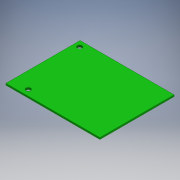
# Autodesk Inventor part: モタドラ
Saved by Autodesk Inventor 2018 (Build 220112000, 112)
## iProperties
Created: 2018-08-16
Part Number: モタドラ
Material: 一般
Document SubType Name: Modeling
Designer: shun2
Density: 1 g/cm^3
Appearance: 濃い緑
Author: shun2
Autodesk Inventor part; units mm, degrees
(part 1 of 2)
ref_plane "YZ Plane" through (0, 0, 0) normal (1, 0, 0) x (0, 1, 0)
ref_plane "XZ Plane" through (0, 0, 0) normal (0, 1, 0) x (-1, 0, 0)
ref_plane "XY Plane" through (0, 0, 0) normal (0, 0, 1) x (1, 0, 0)
sketch "スケッチ1" plane through (0, 0, 0) normal (0, 0, 1) x (1, 0, 0)
  line L0 (65.024, -2.794) -> (65.024, -0.3175)
  line L1 (0, -2.794) -> (0, -0.3175)
  line L2 (37.2085, -2.54) -> (65.024, -2.54)
  line L3 (0, -2.54) -> (27.0027, -2.54)
  line L4 (63.5, -2.032) -> (65.024, -2.54)
  line L5 (63.5, -3.048) -> (65.024, -2.54)
  line L6 (0, -2.54) -> (1.524, -3.048)
  line L7 (0, -2.54) -> (1.524, -2.032)
  line L8 (-2.794, 51.308) -> (-0.3175, 51.308)
  line L9 (-2.794, 0) -> (-0.3175, 0)
  line L10 (-2.54, 30.3505) -> (-2.54, 51.308)
  line L11 (-2.54, 0) -> (-2.54, 20.1447)
  line L12 (-3.048, 49.784) -> (-2.54, 51.308)
  line L13 (-2.54, 51.308) -> (-2.032, 49.784)
  line L14 (-2.54, 0) -> (-2.032, 1.524)
  line L15 (-3.048, 1.524) -> (-2.54, 0)
  line L16 (0, 0) -> (0, 51.308)
  line L17 (0, 51.308) -> (65.024, 51.308)
  line L18 (65.024, 0) -> (65.024, 51.308)
  line L19 (0, 0) -> (65.024, 0)
  line L20 (2.2225, 47.244) -> (5.3975, 47.244)
  line L21 (3.81, 45.6565) -> (3.81, 48.8315)
  line L22 (9.8425, 4.064) -> (13.0175, 4.064)
  line L23 (11.43, 2.4765) -> (11.43, 5.6515)
  line L24 (1.016, 24.384) -> (2.032, 24.384)
  line L25 (1.524, 23.876) -> (1.524, 24.892)
  line L26 (1.016, 21.844) -> (2.032, 21.844)
  line L27 (1.524, 21.336) -> (1.524, 22.352)
  line L28 (1.016, 19.304) -> (2.032, 19.304)
  line L29 (1.524, 18.796) -> (1.524, 19.812)
  line L30 (1.016, 16.764) -> (2.032, 16.764)
  line L31 (1.524, 16.256) -> (1.524, 17.272)
  line L32 (1.016, 14.224) -> (2.032, 14.224)
  line L33 (1.524, 13.716) -> (1.524, 14.732)
  line L34 (1.016, 32.004) -> (2.032, 32.004)
  line L35 (1.524, 31.496) -> (1.524, 32.512)
  line L36 (1.016, 29.464) -> (2.032, 29.464)
  line L37 (1.524, 28.956) -> (1.524, 29.972)
  line L38 (1.016, 26.924) -> (2.032, 26.924)
  line L39 (1.524, 26.416) -> (1.524, 27.432)
  line L40 (1.016, 1.524) -> (2.032, 1.524)
  line L41 (1.524, 1.016) -> (1.524, 2.032)
  line L42 (1.016, 4.064) -> (2.032, 4.064)
  line L43 (1.524, 3.556) -> (1.524, 4.572)
  line L44 (1.016, 6.604) -> (2.032, 6.604)
  line L45 (1.524, 6.096) -> (1.524, 7.112)
  line L46 (1.016, 9.144) -> (2.032, 9.144)
  line L47 (1.524, 8.636) -> (1.524, 9.652)
  line L48 (1.016, 11.684) -> (2.032, 11.684)
  line L49 (1.524, 11.176) -> (1.524, 12.192)
  line L50 (8.382, 47.244) -> (9.398, 47.244)
  line L51 (8.89, 46.736) -> (8.89, 47.752)
  line L52 (8.382, 44.704) -> (9.398, 44.704)
  line L53 (8.89, 44.196) -> (8.89, 45.212)
  line L54 (10.922, 47.244) -> (11.938, 47.244)
  line L55 (11.43, 46.736) -> (11.43, 47.752)
  line L56 (10.922, 44.704) -> (11.938, 44.704)
  line L57 (11.43, 44.196) -> (11.43, 45.212)
  line L58 (13.462, 47.244) -> (14.478, 47.244)
  line L59 (13.97, 46.736) -> (13.97, 47.752)
  line L60 (13.462, 44.704) -> (14.478, 44.704)
  line L61 (13.97, 44.196) -> (13.97, 45.212)
  line L62 (16.002, 47.244) -> (17.018, 47.244)
  line L63 (16.51, 46.736) -> (16.51, 47.752)
  line L64 (16.002, 44.704) -> (17.018, 44.704)
  line L65 (16.51, 44.196) -> (16.51, 45.212)
  line L66 (10.922, 39.497) -> (11.938, 39.497)
  line L67 (11.43, 38.989) -> (11.43, 40.005)
  line L68 (10.922, 36.957) -> (11.938, 36.957)
  line L69 (11.43, 36.449) -> (11.43, 37.465)
  line L70 (13.462, 39.497) -> (14.478, 39.497)
  line L71 (13.97, 38.989) -> (13.97, 40.005)
  line L72 (13.462, 36.957) -> (14.478, 36.957)
  line L73 (13.97, 36.449) -> (13.97, 37.465)
  line L74 (16.002, 39.497) -> (17.018, 39.497)
  line L75 (16.51, 38.989) -> (16.51, 40.005)
  line L76 (16.002, 36.957) -> (17.018, 36.957)
  line L77 (16.51, 36.449) -> (16.51, 37.465)
  line L78 (18.542, 39.497) -> (19.558, 39.497)
  line L79 (19.05, 38.989) -> (19.05, 40.005)
  line L80 (18.542, 36.957) -> (19.558, 36.957)
  line L81 (19.05, 36.449) -> (19.05, 37.465)
  line L82 (19.431, 5.207) -> (20.447, 5.207)
  line L83 (19.939, 4.699) -> (19.939, 5.715)
  line L84 (19.431, 10.2057) -> (20.447, 10.2057)
  line L85 (19.939, 9.7003) -> (19.939, 10.7137)
  line L86 (19.431, 5.207) -> (20.447, 5.207)
  line L87 (19.939, 4.699) -> (19.939, 5.715)
  line L88 (19.431, 8.7071) -> (20.447, 8.7071)
  line L89 (19.939, 8.1991) -> (19.939, 9.2151)
  line L90 (20.066, 14.605) -> (21.082, 14.605)
  line L91 (20.574, 14.097) -> (20.574, 15.113)
  line L92 (22.606, 14.605) -> (23.622, 14.605)
  line L93 (23.114, 14.097) -> (23.114, 15.113)
  line L94 (26.289, 6.858) -> (27.305, 6.858)
  line L95 (26.797, 6.35) -> (26.797, 7.366)
  line L96 (26.289, 9.398) -> (27.305, 9.398)
  line L97 (26.797, 8.89) -> (26.797, 9.906)
  line L98 (26.289, 16.3347) -> (27.305, 16.3347)
  line L99 (26.797, 15.8267) -> (26.797, 16.8427)
  line L100 (25.781, 36.703) -> (26.797, 36.703)
  line L101 (26.289, 36.195) -> (26.289, 37.211)
  line L102 (23.241, 36.703) -> (24.257, 36.703)
  line L103 (23.749, 36.195) -> (23.749, 37.211)
  line L104 (25.4, 39.624) -> (26.416, 39.624)
  line L105 (25.908, 39.116) -> (25.908, 40.132)
  line L106 (59.4868, 28.1813) -> (61.6712, 28.1813)
  line L107 (60.579, 27.0891) -> (60.579, 29.2735)
  line L108 (59.4868, 23.1826) -> (61.6712, 23.1826)
  line L109 (60.579, 22.0904) -> (60.579, 24.2748)
  line L110 (59.4868, 13.1826) -> (61.6712, 13.1826)
  line L111 (60.579, 12.0904) -> (60.579, 14.2748)
  line L112 (59.4868, 18.1813) -> (61.6712, 18.1813)
  line L113 (60.579, 17.0891) -> (60.579, 19.2735)
  line L114 (59.4868, 33.1826) -> (61.6712, 33.1826)
  line L115 (60.579, 32.0904) -> (60.579, 34.2748)
  line L116 (59.4868, 38.1813) -> (61.6712, 38.1813)
  line L117 (60.579, 37.0891) -> (60.579, 39.2735)
  line L118 (61.976, 19.304) -> (62.992, 19.304)
  line L119 (62.484, 18.796) -> (62.484, 19.812)
  line L120 (61.976, 21.844) -> (62.992, 21.844)
  line L121 (62.484, 21.336) -> (62.484, 22.352)
  line L122 (61.976, 24.384) -> (62.992, 24.384)
  line L123 (62.484, 23.876) -> (62.484, 24.892)
  line L124 (61.976, 26.924) -> (62.992, 26.924)
  line L125 (62.484, 26.416) -> (62.484, 27.432)
  line L126 (61.976, 39.624) -> (62.992, 39.624)
  line L127 (62.484, 39.116) -> (62.484, 40.132)
  line L128 (61.976, 37.084) -> (62.992, 37.084)
  line L129 (62.484, 36.576) -> (62.484, 37.592)
  line L130 (61.976, 34.544) -> (62.992, 34.544)
  line L131 (62.484, 34.036) -> (62.484, 35.052)
  line L132 (61.976, 32.004) -> (62.992, 32.004)
  line L133 (62.484, 31.496) -> (62.484, 32.512)
  line L134 (61.976, 29.464) -> (62.992, 29.464)
  line L135 (62.484, 28.956) -> (62.484, 29.972)
  line L136 (61.976, 16.764) -> (62.992, 16.764)
  line L137 (62.484, 16.256) -> (62.484, 17.272)
  line L138 (61.976, 14.224) -> (62.992, 14.224)
  line L139 (62.484, 13.716) -> (62.484, 14.732)
  line L140 (61.976, 11.684) -> (62.992, 11.684)
  line L141 (62.484, 11.176) -> (62.484, 12.192)
  line L142 (54.61, 4.318) -> (55.626, 4.318)
  line L143 (55.118, 3.81) -> (55.118, 4.826)
  line L144 (54.61, 6.858) -> (55.626, 6.858)
  line L145 (55.118, 6.35) -> (55.118, 7.366)
  line L146 (57.15, 4.318) -> (58.166, 4.318)
  line L147 (57.658, 3.81) -> (57.658, 4.826)
  line L148 (57.15, 6.858) -> (58.166, 6.858)
  line L149 (57.658, 6.35) -> (57.658, 7.366)
  line L150 (25.908, 49.784) -> (26.924, 49.784)
  line L151 (26.416, 49.276) -> (26.416, 50.292)
  line L152 (18.288, 49.784) -> (19.304, 49.784)
  line L153 (18.796, 49.276) -> (18.796, 50.292)
  line L154 (28.448, 49.784) -> (29.464, 49.784)
  line L155 (28.956, 49.276) -> (28.956, 50.292)
  line L156 (32.512, 1.524) -> (33.528, 1.524)
  line L157 (33.02, 1.016) -> (33.02, 2.032)
  line L158 (30.988, 49.784) -> (32.004, 49.784)
  line L159 (31.496, 49.276) -> (31.496, 50.292)
  line L160 (33.528, 49.784) -> (34.544, 49.784)
  line L161 (34.036, 49.276) -> (34.036, 50.292)
  line L162 (36.068, 49.784) -> (37.084, 49.784)
  line L163 (36.576, 49.276) -> (36.576, 50.292)
  line L164 (38.608, 49.784) -> (39.624, 49.784)
  line L165 (39.116, 49.276) -> (39.116, 50.292)
  line L166 (41.148, 49.784) -> (42.164, 49.784)
  line L167 (41.656, 49.276) -> (41.656, 50.292)
  line L168 (45.212, 49.784) -> (46.228, 49.784)
  line L169 (45.72, 49.276) -> (45.72, 50.292)
  line L170 (47.752, 49.784) -> (48.768, 49.784)
  line L171 (48.26, 49.276) -> (48.26, 50.292)
  line L172 (50.292, 49.784) -> (51.308, 49.784)
  line L173 (50.8, 49.276) -> (50.8, 50.292)
  line L174 (52.832, 49.784) -> (53.848, 49.784)
  line L175 (53.34, 49.276) -> (53.34, 50.292)
  line L176 (55.372, 49.784) -> (56.388, 49.784)
  line L177 (55.88, 49.276) -> (55.88, 50.292)
  line L178 (57.912, 49.784) -> (58.928, 49.784)
  line L179 (58.42, 49.276) -> (58.42, 50.292)
  line L180 (60.452, 49.784) -> (61.468, 49.784)
  line L181 (60.96, 49.276) -> (60.96, 50.292)
  line L182 (62.992, 49.784) -> (64.008, 49.784)
  line L183 (63.5, 49.276) -> (63.5, 50.292)
  line L184 (35.052, 1.524) -> (36.068, 1.524)
  line L185 (35.56, 1.016) -> (35.56, 2.032)
  line L186 (37.592, 1.524) -> (38.608, 1.524)
  line L187 (38.1, 1.016) -> (38.1, 2.032)
  line L188 (40.132, 1.524) -> (41.148, 1.524)
  line L189 (40.64, 1.016) -> (40.64, 2.032)
  line L190 (42.672, 1.524) -> (43.688, 1.524)
  line L191 (43.18, 1.016) -> (43.18, 2.032)
  line L192 (45.212, 1.524) -> (46.228, 1.524)
  line L193 (45.72, 1.016) -> (45.72, 2.032)
  line L194 (50.292, 1.524) -> (51.308, 1.524)
  line L195 (50.8, 1.016) -> (50.8, 2.032)
  line L196 (52.832, 1.524) -> (53.848, 1.524)
  line L197 (53.34, 1.016) -> (53.34, 2.032)
  line L198 (55.372, 1.524) -> (56.388, 1.524)
  line L199 (55.88, 1.016) -> (55.88, 2.032)
  line L200 (57.912, 1.524) -> (58.928, 1.524)
  line L201 (58.42, 1.016) -> (58.42, 2.032)
  line L202 (60.452, 1.524) -> (61.468, 1.524)
  line L203 (60.96, 1.016) -> (60.96, 2.032)
  line L204 (62.992, 1.524) -> (64.008, 1.524)
  line L205 (63.5, 1.016) -> (63.5, 2.032)
  line L206 (23.368, 49.784) -> (24.384, 49.784)
  line L207 (23.876, 49.276) -> (23.876, 50.292)
  line L208 (20.828, 49.784) -> (21.844, 49.784)
  line L209 (21.336, 49.276) -> (21.336, 50.292)
  line L210 (27.432, 1.524) -> (28.448, 1.524)
  line L211 (27.94, 1.016) -> (27.94, 2.032)
  line L212 (29.972, 1.524) -> (30.988, 1.524)
  line L213 (30.48, 1.016) -> (30.48, 2.032)
  line L214 (49.3395, 25.654) -> (49.7205, 25.654)
  line L215 (49.53, 25.4635) -> (49.53, 25.8445)
  line L216 (50.7365, 25.654) -> (51.1175, 25.654)
  line L217 (50.927, 25.4635) -> (50.927, 25.8445)
  line L218 (49.8475, 26.416) -> (50.2285, 26.416)
  line L219 (50.038, 26.2255) -> (50.038, 26.6065)
  line L220 (48.8315, 26.416) -> (49.2125, 26.416)
  line L221 (49.022, 26.2255) -> (49.022, 26.6065)
  line L222 (48.3235, 25.654) -> (48.7045, 25.654)
  line L223 (48.514, 25.4635) -> (48.514, 25.8445)
  line L224 (29.0195, 35.4813) -> (29.4005, 35.4813)
  line L225 (29.21, 35.2908) -> (29.21, 35.6718)
  line L226 (38.9255, 33.528) -> (39.3065, 33.528)
  line L227 (39.116, 33.3375) -> (39.116, 33.7185)
  line L228 (25.5905, 27.051) -> (25.9715, 27.051)
  line L229 (25.781, 26.8605) -> (25.781, 27.2415)
  line L230 (28.1305, 26.035) -> (28.5115, 26.035)
  line L231 (28.321, 25.8445) -> (28.321, 26.2255)
  line L232 (28.1305, 27.051) -> (28.5115, 27.051)
  line L233 (28.321, 26.8605) -> (28.321, 27.2415)
  line L234 (27.2415, 22.479) -> (27.6225, 22.479)
  line L235 (27.432, 22.2885) -> (27.432, 22.6695)
  line L236 (28.1305, 28.067) -> (28.5115, 28.067)
  line L237 (28.321, 27.8765) -> (28.321, 28.2575)
  line L238 (6.1595, 12.954) -> (6.5405, 12.954)
  line L239 (6.35, 12.7635) -> (6.35, 13.1445)
  line L240 (2.9591, 28.321) -> (3.3401, 28.321)
  line L241 (3.1496, 28.1305) -> (3.1496, 28.5115)
  line L242 (5.1435, 12.954) -> (5.5245, 12.954)
  line L243 (5.334, 12.7635) -> (5.334, 13.1445)
  line L244 (6.6675, 15.113) -> (7.0485, 15.113)
  line L245 (6.858, 14.9225) -> (6.858, 15.3035)
  line L246 (11.8745, 11.557) -> (12.2555, 11.557)
  line L247 (12.065, 11.3665) -> (12.065, 11.7475)
  line L248 (12.1285, 50.038) -> (12.5095, 50.038)
  line L249 (12.319, 49.8475) -> (12.319, 50.2285)
  line L250 (21.1455, 41.402) -> (21.5265, 41.402)
  line L251 (21.336, 41.2115) -> (21.336, 41.5925)
  line L252 (20.259, 43.18) -> (20.64, 43.18)
  line L253 (20.4495, 42.9895) -> (20.4495, 43.3705)
  line L254 (49.8475, 27.94) -> (50.2285, 27.94)
  line L255 (50.038, 27.7495) -> (50.038, 28.1305)
  line L256 (48.8315, 27.94) -> (49.2125, 27.94)
  line L257 (49.022, 27.7495) -> (49.022, 28.1305)
  line L258 (49.8475, 24.892) -> (50.2285, 24.892)
  line L259 (50.038, 24.7015) -> (50.038, 25.0825)
  line L260 (60.6425, 30.226) -> (61.0235, 30.226)
  line L261 (60.833, 30.0355) -> (60.833, 30.4165)
  line L262 (59.1185, 30.226) -> (59.4995, 30.226)
  line L263 (59.309, 30.0355) -> (59.309, 30.4165)
  line L264 (26.858, 43.18) -> (27.239, 43.18)
  line L265 (27.0485, 42.9895) -> (27.0485, 43.3705)
  line L266 (25.2095, 43.18) -> (25.5905, 43.18)
  line L267 (25.4, 42.9895) -> (25.4, 43.3705)
  line L268 (11.3411, 12.1666) -> (11.7221, 12.1666)
  line L269 (11.5316, 11.9761) -> (11.5316, 12.3571)
  line L270 (17.0815, 3.937) -> (17.4625, 3.937)
  line L271 (17.272, 3.7465) -> (17.272, 4.1275)
  line L272 (17.0815, 5.461) -> (17.4625, 5.461)
  line L273 (17.272, 5.2705) -> (17.272, 5.6515)
  line L274 (18.0975, 4.699) -> (18.4785, 4.699)
  line L275 (18.288, 4.5085) -> (18.288, 4.8895)
  line L276 (18.0975, 3.175) -> (18.4785, 3.175)
  line L277 (18.288, 2.9845) -> (18.288, 3.3655)
  line L278 (22.5425, 4.318) -> (22.9235, 4.318)
  line L279 (22.733, 4.1275) -> (22.733, 4.5085)
  line L280 (21.9075, 5.842) -> (22.2885, 5.842)
  line L281 (22.098, 5.6515) -> (22.098, 6.0325)
  line L282 (23.9395, 4.953) -> (24.3205, 4.953)
  line L283 (24.13, 4.7625) -> (24.13, 5.1435)
  line L284 (21.9075, 11.176) -> (22.2885, 11.176)
  line L285 (22.098, 10.9855) -> (22.098, 11.3665)
  line L286 (23.5585, 10.033) -> (23.9395, 10.033)
  line L287 (23.749, 9.8425) -> (23.749, 10.2235)
  line L288 (23.5585, 8.89) -> (23.9395, 8.89)
  line L289 (23.749, 8.6995) -> (23.749, 9.0805)
  line L290 (23.5585, 7.747) -> (23.9395, 7.747)
  line L291 (23.749, 7.5565) -> (23.749, 7.9375)
  line L292 (18.8595, 7.493) -> (19.2405, 7.493)
  line L293 (19.05, 7.3025) -> (19.05, 7.6835)
  line L294 (18.2245, 8.382) -> (18.6055, 8.382)
  line L295 (18.415, 8.1915) -> (18.415, 8.5725)
  line L296 (28.0797, 11.303) -> (28.4607, 11.303)
  line L297 (28.2702, 11.1125) -> (28.2702, 11.4935)
  line L298 (8.6995, 27.051) -> (9.0805, 27.051)
  line L299 (8.89, 26.8605) -> (8.89, 27.2415)
  line L300 (23.8125, 42.164) -> (24.1935, 42.164)
  line L301 (24.003, 41.9735) -> (24.003, 42.3545)
  line L302 (23.8125, 43.18) -> (24.1935, 43.18)
  line L303 (24.003, 42.9895) -> (24.003, 43.3705)
  line L304 (23.8125, 44.196) -> (24.1935, 44.196)
  line L305 (24.003, 44.0055) -> (24.003, 44.3865)
  line L306 (23.8125, 45.212) -> (24.1935, 45.212)
  line L307 (24.003, 45.0215) -> (24.003, 45.4025)
  line L308 (19.7485, 3.175) -> (20.1295, 3.175)
  line L309 (19.939, 2.9845) -> (19.939, 3.3655)
  line L310 (6.5151, 43.8658) -> (6.8961, 43.8658)
  line L311 (6.7056, 43.6753) -> (6.7056, 44.0563)
  line L312 (1.1303, 37.9222) -> (1.5113, 37.9222)
  line L313 (1.3208, 37.7317) -> (1.3208, 38.1127)
  line L314 (7.3279, 41.402) -> (7.7089, 41.402)
  line L315 (7.5184, 41.2115) -> (7.5184, 41.5925)
  line L316 (16.7005, 43.053) -> (17.0815, 43.053)
  line L317 (16.891, 42.8625) -> (16.891, 43.2435)
  line L318 (7.6835, 19.304) -> (8.0645, 19.304)
  line L319 (7.874, 19.1135) -> (7.874, 19.4945)
  line L320 (8.1915, 21.59) -> (8.5725, 21.59)
  line L321 (8.382, 21.3995) -> (8.382, 21.7805)
  line L322 (9.5885, 25.527) -> (9.9695, 25.527)
  line L323 (9.779, 25.3365) -> (9.779, 25.7175)
  line L324 (6.1595, 20.8788) -> (6.5405, 20.8788)
  line L325 (6.35, 20.6883) -> (6.35, 21.0693)
  line L326 (7.5565, 23.622) -> (7.9375, 23.622)
  line L327 (7.747, 23.4315) -> (7.747, 23.8125)
  line L328 (11.811, 27.2288) -> (12.319, 27.2288)
  line L329 (12.065, 26.9748) -> (12.065, 27.4828)
  line L330 (11.2268, 26.416) -> (11.7348, 26.416)
  line L331 (11.4808, 26.162) -> (11.4808, 26.67)
  line L332 (17.3355, 20.193) -> (17.7165, 20.193)
  line L333 (17.526, 20.0025) -> (17.526, 20.3835)
  line L334 (12.8905, 21.971) -> (13.2715, 21.971)
  line L335 (13.081, 21.7805) -> (13.081, 22.1615)
  line L336 (13.7795, 21.209) -> (14.1605, 21.209)
  line L337 (13.97, 21.0185) -> (13.97, 21.3995)
  line L338 (6.9215, 2.667) -> (7.3025, 2.667)
  line L339 (7.112, 2.4765) -> (7.112, 2.8575)
  line L340 (4.1275, 2.667) -> (4.5085, 2.667)
  line L341 (4.318, 2.4765) -> (4.318, 2.8575)
  line L342 (8.6995, 10.287) -> (9.0805, 10.287)
  line L343 (8.89, 10.0965) -> (8.89, 10.4775)
  line L344 (9.4615, 9.144) -> (9.8425, 9.144)
  line L345 (9.652, 8.9535) -> (9.652, 9.3345)
  line L346 (63.5381, 18.034) -> (63.9191, 18.034)
  line L347 (63.7286, 17.8435) -> (63.7286, 18.2245)
  line L348 (63.5635, 33.274) -> (63.9445, 33.274)
  line L349 (63.754, 33.0835) -> (63.754, 33.4645)
  line L350 (59.6265, 42.164) -> (60.0075, 42.164)
  line L351 (59.817, 41.9735) -> (59.817, 42.3545)
  line L352 (13.1445, 16.383) -> (13.5255, 16.383)
  line L353 (13.335, 16.1925) -> (13.335, 16.5735)
  line L354 (25.8445, 31.75) -> (26.2255, 31.75)
  line L355 (26.035, 31.5595) -> (26.035, 31.9405)
  line L356 (14.1605, 35.179) -> (14.5415, 35.179)
  line L357 (14.351, 34.9885) -> (14.351, 35.3695)
  line L358 (23.6855, 17.018) -> (24.0665, 17.018)
  line L359 (23.876, 16.8275) -> (23.876, 17.2085)
  line L360 (11.7475, 19.304) -> (12.1285, 19.304)
  line L361 (11.938, 19.1135) -> (11.938, 19.4945)
  line L362 (29.0703, 11.303) -> (29.4513, 11.303)
  line L363 (29.2608, 11.1125) -> (29.2608, 11.4935)
  line L364 (22.1615, 34.798) -> (22.5425, 34.798)
  line L365 (22.352, 34.6075) -> (22.352, 34.9885)
  line L366 (28.7655, 15.367) -> (29.1465, 15.367)
  line L367 (28.956, 15.1765) -> (28.956, 15.5575)
  line L368 (28.3845, 39.497) -> (28.7655, 39.497)
  line L369 (28.575, 39.3065) -> (28.575, 39.6875)
  line L370 (31.496, 32.4815) -> (32.004, 32.4815)
  line L371 (31.75, 32.2275) -> (31.75, 32.7355)
  line L372 (25.5905, 24.765) -> (25.9715, 24.765)
  line L373 (25.781, 24.5745) -> (25.781, 24.9555)
  line L374 (20.7645, 16.256) -> (21.1455, 16.256)
  line L375 (20.955, 16.0655) -> (20.955, 16.4465)
  line L376 (20.5105, 26.797) -> (20.8915, 26.797)
  line L377 (20.701, 26.6065) -> (20.701, 26.9875)
  line L378 (51.1175, 5.08) -> (51.4985, 5.08)
  line L379 (51.308, 4.8895) -> (51.308, 5.2705)
  line L380 (11.7475, 33.147) -> (12.1285, 33.147)
  line L381 (11.938, 32.9565) -> (11.938, 33.3375)
  line L382 (13.5255, 28.448) -> (13.9065, 28.448)
  line L383 (13.716, 28.2575) -> (13.716, 28.6385)
  line L384 (47.8155, 24.892) -> (48.1965, 24.892)
  line L385 (48.006, 24.7015) -> (48.006, 25.0825)
  line L386 (48.8315, 24.892) -> (49.2125, 24.892)
  line L387 (49.022, 24.7015) -> (49.022, 25.0825)
  line L388 (47.8155, 26.416) -> (48.1965, 26.416)
  line L389 (48.006, 26.2255) -> (48.006, 26.6065)
  line L390 (48.3235, 27.178) -> (48.7045, 27.178)
  line L391 (48.514, 26.9875) -> (48.514, 27.3685)
  line L392 (49.3395, 27.178) -> (49.7205, 27.178)
  line L393 (49.53, 26.9875) -> (49.53, 27.3685)
  line L394 (26.8605, 26.035) -> (27.2415, 26.035)
  line L395 (27.051, 25.8445) -> (27.051, 26.2255)
  line L396 (25.5905, 26.035) -> (25.9715, 26.035)
  line L397 (25.781, 25.8445) -> (25.781, 26.2255)
  line L398 (26.8605, 27.051) -> (27.2415, 27.051)
  line L399 (27.051, 26.8605) -> (27.051, 27.2415)
  line L400 (26.8605, 28.067) -> (27.2415, 28.067)
  line L401 (27.051, 27.8765) -> (27.051, 28.2575)
  line L402 (25.5905, 28.067) -> (25.9715, 28.067)
  line L403 (25.781, 27.8765) -> (25.781, 28.2575)
  line L404 (27.2415, 24.765) -> (27.6225, 24.765)
  line L405 (27.432, 24.5745) -> (27.432, 24.9555)
  line L406 (26.3525, 23.495) -> (26.7335, 23.495)
  line L407 (26.543, 23.3045) -> (26.543, 23.6855)
  line L408 (24.8285, 22.733) -> (25.2095, 22.733)
  line L409 (25.019, 22.5425) -> (25.019, 22.9235)
  line L410 (23.9395, 24.765) -> (24.3205, 24.765)
  line L411 (24.13, 24.5745) -> (24.13, 24.9555)
  line L412 (23.9395, 28.067) -> (24.3205, 28.067)
  line L413 (24.13, 27.8765) -> (24.13, 28.2575)
  line L414 (23.9395, 26.416) -> (24.3205, 26.416)
  line L415 (24.13, 26.2255) -> (24.13, 26.6065)
  line L416 (49.784, 40.513) -> (50.292, 40.513)
  line L417 (50.038, 40.259) -> (50.038, 40.767)
  line L418 (49.784, 41.402) -> (50.292, 41.402)
  line L419 (50.038, 41.148) -> (50.038, 41.656)
  line L420 (49.784, 46.609) -> (50.292, 46.609)
  line L421 (50.038, 46.355) -> (50.038, 46.863)
  line L422 (49.784, 32.512) -> (50.292, 32.512)
  line L423 (50.038, 32.258) -> (50.038, 32.766)
  line L424 (49.784, 37.465) -> (50.292, 37.465)
  line L425 (50.038, 37.211) -> (50.038, 37.719)
  line L426 (49.784, 38.354) -> (50.292, 38.354)
  line L427 (50.038, 38.1) -> (50.038, 38.608)
  line L428 (49.784, 15.367) -> (50.292, 15.367)
  line L429 (50.038, 15.113) -> (50.038, 15.621)
  line L430 (49.784, 16.256) -> (50.292, 16.256)
  line L431 (50.038, 16.002) -> (50.038, 16.51)
  line L432 (49.784, 21.336) -> (50.292, 21.336)
  line L433 (50.038, 21.082) -> (50.038, 21.59)
  line L434 (49.784, 12.319) -> (50.292, 12.319)
  line L435 (50.038, 12.065) -> (50.038, 12.573)
  line L436 (49.784, 13.335) -> (50.292, 13.335)
  line L437 (50.038, 13.081) -> (50.038, 13.589)
  line L438 (49.784, 7.366) -> (50.292, 7.366)
  line L439 (50.038, 7.112) -> (50.038, 7.62)
  line L440 (7.5565, 50.038) -> (7.9375, 50.038)
  line L441 (7.747, 49.8475) -> (7.747, 50.2285)
  line L442 (30.0355, 6.096) -> (30.4165, 6.096)
  line L443 (30.226, 5.9055) -> (30.226, 6.2865)
  line L444 (31.3055, 6.096) -> (31.6865, 6.096)
  line L445 (31.496, 5.9055) -> (31.496, 6.2865)
  line L446 (32.5755, 6.096) -> (32.9565, 6.096)
  line L447 (32.766, 5.9055) -> (32.766, 6.2865)
  line L448 (33.8455, 6.096) -> (34.2265, 6.096)
  line L449 (34.036, 5.9055) -> (34.036, 6.2865)
  line L450 (35.1155, 6.096) -> (35.4965, 6.096)
  line L451 (35.306, 5.9055) -> (35.306, 6.2865)
  line L452 (36.3855, 6.096) -> (36.7665, 6.096)
  line L453 (36.576, 5.9055) -> (36.576, 6.2865)
  line L454 (37.6555, 6.096) -> (38.0365, 6.096)
  line L455 (37.846, 5.9055) -> (37.846, 6.2865)
  line L456 (38.9255, 6.096) -> (39.3065, 6.096)
  line L457 (39.116, 5.9055) -> (39.116, 6.2865)
  line L458 (40.1955, 6.096) -> (40.5765, 6.096)
  line L459 (40.386, 5.9055) -> (40.386, 6.2865)
  line L460 (41.4655, 6.096) -> (41.8465, 6.096)
  line L461 (41.656, 5.9055) -> (41.656, 6.2865)
  line L462 (42.7355, 6.096) -> (43.1165, 6.096)
  line L463 (42.926, 5.9055) -> (42.926, 6.2865)
  line L464 (44.0055, 6.096) -> (44.3865, 6.096)
  line L465 (44.196, 5.9055) -> (44.196, 6.2865)
  line L466 (45.2755, 6.096) -> (45.6565, 6.096)
  line L467 (45.466, 5.9055) -> (45.466, 6.2865)
  line L468 (46.5455, 6.096) -> (46.9265, 6.096)
  line L469 (46.736, 5.9055) -> (46.736, 6.2865)
  line L470 (47.8155, 6.096) -> (48.1965, 6.096)
  line L471 (48.006, 5.9055) -> (48.006, 6.2865)
  line L472 (49.0855, 6.096) -> (49.4665, 6.096)
  line L473 (49.276, 5.9055) -> (49.276, 6.2865)
  line L474 (50.3555, 6.096) -> (50.7365, 6.096)
  line L475 (50.546, 5.9055) -> (50.546, 6.2865)
  line L476 (45.7835, 5.08) -> (46.1645, 5.08)
  line L477 (45.974, 4.8895) -> (45.974, 5.2705)
  line L478 (47.0535, 5.08) -> (47.4345, 5.08)
  line L479 (47.244, 4.8895) -> (47.244, 5.2705)
  line L480 (48.3235, 5.08) -> (48.7045, 5.08)
  line L481 (48.514, 4.8895) -> (48.514, 5.2705)
  line L482 (49.5935, 5.08) -> (49.9745, 5.08)
  line L483 (49.784, 4.8895) -> (49.784, 5.2705)
  line L484 (20.5105, 25.908) -> (20.8915, 25.908)
  line L485 (20.701, 25.7175) -> (20.701, 26.0985)
  line L486 (20.5105, 24.892) -> (20.8915, 24.892)
  line L487 (20.701, 24.7015) -> (20.701, 25.0825)
  line L488 (22.0345, 24.003) -> (22.4155, 24.003)
  line L489 (22.225, 23.8125) -> (22.225, 24.1935)
  line L490 (22.0345, 23.114) -> (22.4155, 23.114)
  line L491 (22.225, 22.9235) -> (22.225, 23.3045)
  line L492 (22.0345, 22.225) -> (22.4155, 22.225)
  line L493 (22.225, 22.0345) -> (22.225, 22.4155)
  line L494 (20.5105, 27.686) -> (20.8915, 27.686)
  line L495 (20.701, 27.4955) -> (20.701, 27.8765)
  line L496 (52.0065, 26.924) -> (52.3875, 26.924)
  line L497 (52.197, 26.7335) -> (52.197, 27.1145)
  line L498 (52.0065, 28.067) -> (52.3875, 28.067)
  line L499 (52.197, 27.8765) -> (52.197, 28.2575)
  line L500 (31.4731, 36.482) -> (31.8541, 36.482)
  line L501 (31.6636, 36.2915) -> (31.6636, 36.6725)
  line L502 (19.3675, 43.18) -> (19.7485, 43.18)
  line L503 (19.558, 42.9895) -> (19.558, 43.3705)
  line L504 (21.6535, 43.18) -> (22.0345, 43.18)
  line L505 (21.844, 42.9895) -> (21.844, 43.3705)
  line L506 (19.6215, 41.402) -> (20.0025, 41.402)
  line L507 (19.812, 41.2115) -> (19.812, 41.5925)
  line L508 (28.702, 44.831) -> (29.21, 44.831)
  line L509 (28.956, 44.577) -> (28.956, 45.085)
  line L510 (13.5509, 29.2354) -> (13.9319, 29.2354)
  line L511 (13.7414, 29.0449) -> (13.7414, 29.4259)
  line L512 (12.6619, 33.1724) -> (13.0429, 33.1724)
  line L513 (12.8524, 32.9819) -> (12.8524, 33.3629)
  line L514 (16.7005, 21.336) -> (17.0815, 21.336)
  line L515 (16.891, 21.1455) -> (16.891, 21.5265)
  line L516 (23.6855, 3.175) -> (24.0665, 3.175)
  line L517 (23.876, 2.9845) -> (23.876, 3.3655)
  line L518 (25.2095, 5.842) -> (25.5905, 5.842)
  line L519 (25.4, 5.6515) -> (25.4, 6.0325)
  line L520 (21.3995, 3.175) -> (21.7805, 3.175)
  line L521 (21.59, 2.9845) -> (21.59, 3.3655)
  line L522 (57.9755, 29.718) -> (58.3565, 29.718)
  line L523 (58.166, 29.5275) -> (58.166, 29.9085)
  line L524 (55.9435, 31.115) -> (56.3245, 31.115)
  line L525 (56.134, 30.9245) -> (56.134, 31.3055)
  line L526 (54.4195, 31.115) -> (54.8005, 31.115)
  line L527 (54.61, 30.9245) -> (54.61, 31.3055)
  line L528 (53.1495, 31.115) -> (53.5305, 31.115)
  line L529 (53.34, 30.9245) -> (53.34, 31.3055)
  line L530 (57.9755, 27.305) -> (58.3565, 27.305)
  line L531 (58.166, 27.1145) -> (58.166, 27.4955)
  line L532 (57.0865, 27.94) -> (57.4675, 27.94)
  line L533 (57.277, 27.7495) -> (57.277, 28.1305)
  line L534 (60.7695, 26.162) -> (61.1505, 26.162)
  line L535 (60.96, 25.9715) -> (60.96, 26.3525)
  line L536 (63.5635, 29.972) -> (63.9445, 29.972)
  line L537 (63.754, 29.7815) -> (63.754, 30.1625)
  line L538 (63.5635, 28.956) -> (63.9445, 28.956)
  line L539 (63.754, 28.7655) -> (63.754, 29.1465)
  line L540 (63.5635, 27.432) -> (63.9445, 27.432)
  line L541 (63.754, 27.2415) -> (63.754, 27.6225)
  line L542 (63.5635, 26.162) -> (63.9445, 26.162)
  line L543 (63.754, 25.9715) -> (63.754, 26.3525)
  line L544 (21.9075, 7.747) -> (22.2885, 7.747)
  line L545 (22.098, 7.5565) -> (22.098, 7.9375)
  line L546 (21.9075, 8.89) -> (22.2885, 8.89)
  line L547 (22.098, 8.6995) -> (22.098, 9.0805)
  line L548 (21.9075, 10.033) -> (22.2885, 10.033)
  line L549 (22.098, 9.8425) -> (22.098, 10.2235)
  line L550 (25.0825, 10.541) -> (25.4635, 10.541)
  line L551 (25.273, 10.3505) -> (25.273, 10.7315)
  line L552 (25.0825, 8.255) -> (25.4635, 8.255)
  line L553 (25.273, 8.0645) -> (25.273, 8.4455)
  line L554 (51.6255, 6.096) -> (52.0065, 6.096)
  line L555 (51.816, 5.9055) -> (51.816, 6.2865)
  line L556 (52.3875, 5.08) -> (52.7685, 5.08)
  line L557 (52.578, 4.8895) -> (52.578, 5.2705)
  line L558 (52.8955, 6.096) -> (53.2765, 6.096)
  line L559 (53.086, 5.9055) -> (53.086, 6.2865)
  line L560 (32.004, 44.831) -> (32.512, 44.831)
  line L561 (32.258, 44.577) -> (32.258, 45.085)
  line L562 (28.956, 8.382) -> (29.464, 8.382)
  line L563 (29.21, 8.128) -> (29.21, 8.636)
  line L564 (31.623, 21.336) -> (32.131, 21.336)
  line L565 (31.877, 21.082) -> (31.877, 21.59)
  line L566 (28.829, 21.336) -> (29.337, 21.336)
  line L567 (29.083, 21.082) -> (29.083, 21.59)
  line L568 (28.9052, 32.4815) -> (29.4132, 32.4815)
  line L569 (29.1592, 32.2275) -> (29.1592, 32.7355)
  line L570 (31.7119, 9.525) -> (32.2199, 9.525)
  line L571 (31.9659, 9.271) -> (31.9659, 9.779)
  line L572 (31.75, 8.509) -> (32.258, 8.509)
  line L573 (32.004, 8.255) -> (32.004, 8.763)
  line L574 (62.6745, 9.271) -> (63.0555, 9.271)
  line L575 (62.865, 9.0805) -> (62.865, 9.4615)
  line L576 (46.228, 7.874) -> (46.736, 7.874)
  line L577 (46.482, 7.62) -> (46.482, 8.128)
  line L578 (46.228, 9.398) -> (46.736, 9.398)
  line L579 (46.482, 9.144) -> (46.482, 9.652)
  line L580 (46.228, 10.922) -> (46.736, 10.922)
  line L581 (46.482, 10.668) -> (46.482, 11.176)
  line L582 (46.228, 12.446) -> (46.736, 12.446)
  line L583 (46.482, 12.192) -> (46.482, 12.7)
  line L584 (46.228, 20.8458) -> (46.736, 20.8458)
  line L585 (46.482, 20.5918) -> (46.482, 21.0998)
  line L586 (46.228, 19.3218) -> (46.736, 19.3218)
  line L587 (46.482, 19.0678) -> (46.482, 19.5758)
  line L588 (46.228, 17.7978) -> (46.736, 17.7978)
  line L589 (46.482, 17.5438) -> (46.482, 18.0518)
  line L590 (46.228, 16.2738) -> (46.736, 16.2738)
  line L591 (46.482, 16.0198) -> (46.482, 16.5278)
  line L592 (46.228, 37.592) -> (46.736, 37.592)
  line L593 (46.482, 37.338) -> (46.482, 37.846)
  line L594 (46.228, 36.068) -> (46.736, 36.068)
  line L595 (46.482, 35.814) -> (46.482, 36.322)
  line L596 (46.228, 34.544) -> (46.736, 34.544)
  line L597 (46.482, 34.29) -> (46.482, 34.798)
  line L598 (46.228, 33.02) -> (46.736, 33.02)
  line L599 (46.482, 32.766) -> (46.482, 33.274)
  line L600 (46.228, 45.9918) -> (46.736, 45.9918)
  line L601 (46.482, 45.7378) -> (46.482, 46.2458)
  line L602 (46.228, 44.4678) -> (46.736, 44.4678)
  line L603 (46.482, 44.2138) -> (46.482, 44.7218)
  line L604 (46.228, 42.9438) -> (46.736, 42.9438)
  line L605 (46.482, 42.6898) -> (46.482, 43.1978)
  line L606 (46.228, 41.4198) -> (46.736, 41.4198)
  line L607 (46.482, 41.1658) -> (46.482, 41.6738)
  line L608 (32.258, 11.43) -> (32.766, 11.43)
  line L609 (32.512, 11.176) -> (32.512, 11.684)
  line L610 (32.258, 13.208) -> (32.766, 13.208)
  line L611 (32.512, 12.954) -> (32.512, 13.462)
  line L612 (32.258, 14.986) -> (32.766, 14.986)
  line L613 (32.512, 14.732) -> (32.512, 15.24)
  line L614 (32.258, 16.764) -> (32.766, 16.764)
  line L615 (32.512, 16.51) -> (32.512, 17.018)
  line L616 (32.258, 18.542) -> (32.766, 18.542)
  line L617 (32.512, 18.288) -> (32.512, 18.796)
  line L618 (32.512, 38.354) -> (33.02, 38.354)
  line L619 (32.766, 38.1) -> (32.766, 38.608)
  line L620 (32.512, 40.132) -> (33.02, 40.132)
  line L621 (32.766, 39.878) -> (32.766, 40.386)
  line L622 (32.512, 41.91) -> (33.02, 41.91)
  line L623 (32.766, 41.656) -> (32.766, 42.164)
  line L624 (32.512, 43.434) -> (33.02, 43.434)
  line L625 (32.766, 43.18) -> (32.766, 43.688)
  line L626 (32.004, 34.163) -> (32.512, 34.163)
  line L627 (32.258, 33.909) -> (32.258, 34.417)
  line L628 (24.765, 33.782) -> (25.273, 33.782)
  line L629 (25.019, 33.528) -> (25.019, 34.036)
  line L630 (23.495, 33.782) -> (24.003, 33.782)
  line L631 (23.749, 33.528) -> (23.749, 34.036)
  line L632 (57.9755, 28.448) -> (58.3565, 28.448)
  line L633 (58.166, 28.2575) -> (58.166, 28.6385)
  line L634 (56.8325, 29.718) -> (57.2135, 29.718)
  line L635 (57.023, 29.5275) -> (57.023, 29.9085)
  line L636 (40.1904, 43.1419) -> (40.5714, 43.1419)
  line L637 (40.3809, 42.9514) -> (40.3809, 43.3324)
  line L638 (40.1904, 44.2214) -> (40.5714, 44.2214)
  line L639 (40.3809, 44.0309) -> (40.3809, 44.4119)
  line L640 (44.6888, 46.3829) -> (45.0698, 46.3829)
  line L641 (44.8793, 46.1924) -> (44.8793, 46.5734)
  line L642 (43.5635, 46.3829) -> (43.9445, 46.3829)
  line L643 (43.754, 46.1924) -> (43.754, 46.5734)
  line L644 (41.3156, 46.3829) -> (41.6966, 46.3829)
  line L645 (41.5061, 46.1924) -> (41.5061, 46.5734)
  line L646 (40.1904, 45.3009) -> (40.5714, 45.3009)
  line L647 (40.3809, 45.1104) -> (40.3809, 45.4914)
  line L648 (42.4383, 46.3829) -> (42.8193, 46.3829)
  line L649 (42.6288, 46.1924) -> (42.6288, 46.5734)
  line L650 (40.1904, 46.3829) -> (40.5714, 46.3829)
  line L651 (40.3809, 46.1924) -> (40.3809, 46.5734)
  line L652 (40.1904, 42.0624) -> (40.5714, 42.0624)
  line L653 (40.3809, 41.8719) -> (40.3809, 42.2529)
  line L654 (40.1904, 40.9829) -> (40.5714, 40.9829)
  line L655 (40.3809, 40.7924) -> (40.3809, 41.1734)
  line L656 (41.3156, 40.9829) -> (41.6966, 40.9829)
  line L657 (41.5061, 40.7924) -> (41.5061, 41.1734)
  line L658 (41.3156, 42.0624) -> (41.6966, 42.0624)
  line L659 (41.5061, 41.8719) -> (41.5061, 42.2529)
  line L660 (41.3156, 45.3009) -> (41.6966, 45.3009)
  line L661 (41.5061, 45.1104) -> (41.5061, 45.4914)
  line L662 (41.3156, 44.2214) -> (41.6966, 44.2214)
  line L663 (41.5061, 44.0309) -> (41.5061, 44.4119)
  line L664 (41.3156, 43.1419) -> (41.6966, 43.1419)
  line L665 (41.5061, 42.9514) -> (41.5061, 43.3324)
  line L666 (42.4383, 40.9829) -> (42.8193, 40.9829)
  line L667 (42.6288, 40.7924) -> (42.6288, 41.1734)
  line L668 (42.4383, 42.0624) -> (42.8193, 42.0624)
  line L669 (42.6288, 41.8719) -> (42.6288, 42.2529)
  line L670 (42.4383, 45.3009) -> (42.8193, 45.3009)
  line L671 (42.6288, 45.1104) -> (42.6288, 45.4914)
  line L672 (42.4383, 44.2214) -> (42.8193, 44.2214)
  line L673 (42.6288, 44.0309) -> (42.6288, 44.4119)
  line L674 (42.4383, 43.1419) -> (42.8193, 43.1419)
  line L675 (42.6288, 42.9514) -> (42.6288, 43.3324)
  line L676 (43.5635, 40.9829) -> (43.9445, 40.9829)
  line L677 (43.754, 40.7924) -> (43.754, 41.1734)
  line L678 (43.5635, 42.0624) -> (43.9445, 42.0624)
  line L679 (43.754, 41.8719) -> (43.754, 42.2529)
  line L680 (43.5635, 45.3009) -> (43.9445, 45.3009)
  line L681 (43.754, 45.1104) -> (43.754, 45.4914)
  line L682 (43.5635, 44.2214) -> (43.9445, 44.2214)
  line L683 (43.754, 44.0309) -> (43.754, 44.4119)
  line L684 (43.5635, 43.1419) -> (43.9445, 43.1419)
  line L685 (43.754, 42.9514) -> (43.754, 43.3324)
  line L686 (44.6888, 40.9829) -> (45.0698, 40.9829)
  line L687 (44.8793, 40.7924) -> (44.8793, 41.1734)
  line L688 (44.6888, 42.0624) -> (45.0698, 42.0624)
  line L689 (44.8793, 41.8719) -> (44.8793, 42.2529)
  line L690 (44.6888, 45.3009) -> (45.0698, 45.3009)
  line L691 (44.8793, 45.1104) -> (44.8793, 45.4914)
  line L692 (44.6888, 44.2214) -> (45.0698, 44.2214)
  line L693 (44.8793, 44.0309) -> (44.8793, 44.4119)
  line L694 (44.6888, 43.1419) -> (45.0698, 43.1419)
  line L695 (44.8793, 42.9514) -> (44.8793, 43.3324)
  line L696 (44.6888, 35.8216) -> (45.0698, 35.8216)
  line L697 (44.8793, 35.6311) -> (44.8793, 36.0121)
  line L698 (44.6888, 34.7421) -> (45.0698, 34.7421)
  line L699 (44.8793, 34.5516) -> (44.8793, 34.9326)
  line L700 (44.6888, 33.6626) -> (45.0698, 33.6626)
  line L701 (44.8793, 33.4721) -> (44.8793, 33.8531)
  line L702 (44.6888, 36.9011) -> (45.0698, 36.9011)
  line L703 (44.8793, 36.7106) -> (44.8793, 37.0916)
  line L704 (44.6888, 37.9832) -> (45.0698, 37.9832)
  line L705 (44.8793, 37.7927) -> (44.8793, 38.1737)
  line L706 (43.5635, 35.8216) -> (43.9445, 35.8216)
  line L707 (43.754, 35.6311) -> (43.754, 36.0121)
  line L708 (43.5635, 34.7421) -> (43.9445, 34.7421)
  line L709 (43.754, 34.5516) -> (43.754, 34.9326)
  line L710 (43.5635, 33.6626) -> (43.9445, 33.6626)
  line L711 (43.754, 33.4721) -> (43.754, 33.8531)
  line L712 (43.5635, 36.9011) -> (43.9445, 36.9011)
  line L713 (43.754, 36.7106) -> (43.754, 37.0916)
  line L714 (43.5635, 37.9832) -> (43.9445, 37.9832)
  line L715 (43.754, 37.7927) -> (43.754, 38.1737)
  line L716 (42.4383, 35.8216) -> (42.8193, 35.8216)
  line L717 (42.6288, 35.6311) -> (42.6288, 36.0121)
  line L718 (42.4383, 34.7421) -> (42.8193, 34.7421)
  line L719 (42.6288, 34.5516) -> (42.6288, 34.9326)
  line L720 (42.4383, 33.6626) -> (42.8193, 33.6626)
  line L721 (42.6288, 33.4721) -> (42.6288, 33.8531)
  line L722 (42.4383, 36.9011) -> (42.8193, 36.9011)
  line L723 (42.6288, 36.7106) -> (42.6288, 37.0916)
  line L724 (42.4383, 37.9832) -> (42.8193, 37.9832)
  line L725 (42.6288, 37.7927) -> (42.6288, 38.1737)
  line L726 (41.3156, 35.8216) -> (41.6966, 35.8216)
  line L727 (41.5061, 35.6311) -> (41.5061, 36.0121)
  line L728 (41.3156, 34.7421) -> (41.6966, 34.7421)
  line L729 (41.5061, 34.5516) -> (41.5061, 34.9326)
  line L730 (41.3156, 33.6626) -> (41.6966, 33.6626)
  line L731 (41.5061, 33.4721) -> (41.5061, 33.8531)
  line L732 (41.3156, 36.9011) -> (41.6966, 36.9011)
  line L733 (41.5061, 36.7106) -> (41.5061, 37.0916)
  line L734 (41.3156, 37.9832) -> (41.6966, 37.9832)
  line L735 (41.5061, 37.7927) -> (41.5061, 38.1737)
  line L736 (40.1904, 37.9832) -> (40.5714, 37.9832)
  line L737 (40.3809, 37.7927) -> (40.3809, 38.1737)
  line L738 (40.1904, 36.9011) -> (40.5714, 36.9011)
  line L739 (40.3809, 36.7106) -> (40.3809, 37.0916)
  line L740 (40.1904, 32.5831) -> (40.5714, 32.5831)
  line L741 (40.3809, 32.3926) -> (40.3809, 32.7736)
  line L742 (42.4383, 32.5831) -> (42.8193, 32.5831)
  line L743 (42.6288, 32.3926) -> (42.6288, 32.7736)
  line L744 (40.1904, 33.6626) -> (40.5714, 33.6626)
  line L745 (40.3809, 33.4721) -> (40.3809, 33.8531)
  line L746 (41.3156, 32.5831) -> (41.6966, 32.5831)
  line L747 (41.5061, 32.3926) -> (41.5061, 32.7736)
  line L748 (43.5635, 32.5831) -> (43.9445, 32.5831)
  line L749 (43.754, 32.3926) -> (43.754, 32.7736)
  line L750 (44.6888, 32.5831) -> (45.0698, 32.5831)
  line L751 (44.8793, 32.3926) -> (44.8793, 32.7736)
  line L752 (40.1904, 34.7421) -> (40.5714, 34.7421)
  line L753 (40.3809, 34.5516) -> (40.3809, 34.9326)
  line L754 (40.1904, 35.8216) -> (40.5714, 35.8216)
  line L755 (40.3809, 35.6311) -> (40.3809, 36.0121)
  line L756 (38.5902, 40.0558) -> (38.9712, 40.0558)
  line L757 (38.7807, 39.8653) -> (38.7807, 40.2463)
  line L758 (38.5902, 41.1378) -> (38.9712, 41.1378)
  line L759 (38.7807, 40.9473) -> (38.7807, 41.3283)
  line L760 (37.465, 40.0558) -> (37.846, 40.0558)
  line L761 (37.6555, 39.8653) -> (37.6555, 40.2463)
  line L762 (37.465, 41.1378) -> (37.846, 41.1378)
  line L763 (37.6555, 40.9473) -> (37.6555, 41.3283)
  line L764 (36.3398, 40.0558) -> (36.7208, 40.0558)
  line L765 (36.5303, 39.8653) -> (36.5303, 40.2463)
  line L766 (36.3398, 41.1378) -> (36.7208, 41.1378)
  line L767 (36.5303, 40.9473) -> (36.5303, 41.3283)
  line L768 (35.2146, 40.0558) -> (35.5956, 40.0558)
  line L769 (35.4051, 39.8653) -> (35.4051, 40.2463)
  line L770 (35.2146, 41.1378) -> (35.5956, 41.1378)
  line L771 (35.4051, 40.9473) -> (35.4051, 41.3283)
  line L772 (34.0893, 42.2173) -> (34.4703, 42.2173)
  line L773 (34.2798, 42.0268) -> (34.2798, 42.4078)
  line L774 (36.3398, 42.2173) -> (36.7208, 42.2173)
  line L775 (36.5303, 42.0268) -> (36.5303, 42.4078)
  line L776 (34.0893, 41.1378) -> (34.4703, 41.1378)
  line L777 (34.2798, 40.9473) -> (34.2798, 41.3283)
  line L778 (35.2146, 42.2173) -> (35.5956, 42.2173)
  line L779 (35.4051, 42.0268) -> (35.4051, 42.4078)
  line L780 (37.465, 42.2173) -> (37.846, 42.2173)
  line L781 (37.6555, 42.0268) -> (37.6555, 42.4078)
  line L782 (38.5902, 42.2173) -> (38.9712, 42.2173)
  line L783 (38.7807, 42.0268) -> (38.7807, 42.4078)
  line L784 (34.0893, 40.0558) -> (34.4703, 40.0558)
  line L785 (34.2798, 39.8653) -> (34.2798, 40.2463)
  line L786 (34.0893, 38.9077) -> (34.4703, 38.9077)
  line L787 (34.2798, 38.7172) -> (34.2798, 39.0982)
  line L788 (38.5902, 36.7462) -> (38.9712, 36.7462)
  line L789 (38.7807, 36.5557) -> (38.7807, 36.9367)
  line L790 (37.465, 36.7462) -> (37.846, 36.7462)
  line L791 (37.6555, 36.5557) -> (37.6555, 36.9367)
  line L792 (35.2146, 36.7462) -> (35.5956, 36.7462)
  line L793 (35.4051, 36.5557) -> (35.4051, 36.9367)
  line L794 (34.0893, 37.8282) -> (34.4703, 37.8282)
  line L795 (34.2798, 37.6377) -> (34.2798, 38.0187)
  line L796 (36.3398, 36.7462) -> (36.7208, 36.7462)
  line L797 (36.5303, 36.5557) -> (36.5303, 36.9367)
  line L798 (34.0893, 36.7462) -> (34.4703, 36.7462)
  line L799 (34.2798, 36.5557) -> (34.2798, 36.9367)
  line L800 (35.2146, 37.8282) -> (35.5956, 37.8282)
  line L801 (35.4051, 37.6377) -> (35.4051, 38.0187)
  line L802 (35.2146, 38.9077) -> (35.5956, 38.9077)
  line L803 (35.4051, 38.7172) -> (35.4051, 39.0982)
  line L804 (36.3398, 37.8282) -> (36.7208, 37.8282)
  line L805 (36.5303, 37.6377) -> (36.5303, 38.0187)
  line L806 (36.3398, 38.9077) -> (36.7208, 38.9077)
  line L807 (36.5303, 38.7172) -> (36.5303, 39.0982)
  line L808 (37.465, 37.8282) -> (37.846, 37.8282)
  line L809 (37.6555, 37.6377) -> (37.6555, 38.0187)
  line L810 (37.465, 38.9077) -> (37.846, 38.9077)
  line L811 (37.6555, 38.7172) -> (37.6555, 39.0982)
  line L812 (38.5902, 37.8282) -> (38.9712, 37.8282)
  line L813 (38.7807, 37.6377) -> (38.7807, 38.0187)
  line L814 (38.5902, 38.9077) -> (38.9712, 38.9077)
  line L815 (38.7807, 38.7172) -> (38.7807, 39.0982)
  line L816 (38.5902, 35.6667) -> (38.9712, 35.6667)
  line L817 (38.7807, 35.4762) -> (38.7807, 35.8572)
  line L818 (37.465, 35.6667) -> (37.846, 35.6667)
  line L819 (37.6555, 35.4762) -> (37.6555, 35.8572)
  line L820 (36.3398, 35.6667) -> (36.7208, 35.6667)
  line L821 (36.5303, 35.4762) -> (36.5303, 35.8572)
  line L822 (35.2146, 35.6667) -> (35.5956, 35.6667)
  line L823 (35.4051, 35.4762) -> (35.4051, 35.8572)
  line L824 (34.0893, 34.5872) -> (34.4703, 34.5872)
  line L825 (34.2798, 34.3967) -> (34.2798, 34.7777)
  line L826 (36.3398, 34.5872) -> (36.7208, 34.5872)
  line L827 (36.5303, 34.3967) -> (36.5303, 34.7777)
  line L828 (34.0893, 35.6667) -> (34.4703, 35.6667)
  line L829 (34.2798, 35.4762) -> (34.2798, 35.8572)
  line L830 (35.2146, 34.5872) -> (35.5956, 34.5872)
  line L831 (35.4051, 34.3967) -> (35.4051, 34.7777)
  line L832 (37.465, 34.5872) -> (37.846, 34.5872)
  line L833 (37.6555, 34.3967) -> (37.6555, 34.7777)
  line L834 (38.5902, 34.5872) -> (38.9712, 34.5872)
  line L835 (38.7807, 34.3967) -> (38.7807, 34.7777)
  line L836 (38.5902, 44.3763) -> (38.9712, 44.3763)
  line L837 (38.7807, 44.1858) -> (38.7807, 44.5668)
  line L838 (37.465, 44.3763) -> (37.846, 44.3763)
  line L839 (37.6555, 44.1858) -> (37.6555, 44.5668)
  line L840 (35.2146, 44.3763) -> (35.5956, 44.3763)
  line L841 (35.4051, 44.1858) -> (35.4051, 44.5668)
  line L842 (34.0893, 43.2968) -> (34.4703, 43.2968)
  line L843 (34.2798, 43.1063) -> (34.2798, 43.4873)
  line L844 (36.3398, 44.3763) -> (36.7208, 44.3763)
  line L845 (36.5303, 44.1858) -> (36.5303, 44.5668)
  line L846 (34.0893, 44.3763) -> (34.4703, 44.3763)
  line L847 (34.2798, 44.1858) -> (34.2798, 44.5668)
  line L848 (35.2146, 43.2968) -> (35.5956, 43.2968)
  line L849 (35.4051, 43.1063) -> (35.4051, 43.4873)
  line L850 (36.3398, 43.2968) -> (36.7208, 43.2968)
  line L851 (36.5303, 43.1063) -> (36.5303, 43.4873)
  line L852 (37.465, 43.2968) -> (37.846, 43.2968)
  line L853 (37.6555, 43.1063) -> (37.6555, 43.4873)
  line L854 (38.5902, 43.2968) -> (38.9712, 43.2968)
  line L855 (38.7807, 43.1063) -> (38.7807, 43.4873)
  line L856 (40.1904, 17.9959) -> (40.5714, 17.9959)
  line L857 (40.3809, 17.8054) -> (40.3809, 18.1864)
  line L858 (40.1904, 19.0754) -> (40.5714, 19.0754)
  line L859 (40.3809, 18.8849) -> (40.3809, 19.2659)
  line L860 (44.6888, 21.2369) -> (45.0698, 21.2369)
  line L861 (44.8793, 21.0464) -> (44.8793, 21.4274)
  line L862 (43.5635, 21.2369) -> (43.9445, 21.2369)
  line L863 (43.754, 21.0464) -> (43.754, 21.4274)
  line L864 (41.3156, 21.2369) -> (41.6966, 21.2369)
  line L865 (41.5061, 21.0464) -> (41.5061, 21.4274)
  line L866 (40.1904, 20.1549) -> (40.5714, 20.1549)
  line L867 (40.3809, 19.9644) -> (40.3809, 20.3454)
  line L868 (42.4383, 21.2369) -> (42.8193, 21.2369)
  line L869 (42.6288, 21.0464) -> (42.6288, 21.4274)
  line L870 (40.1904, 21.2369) -> (40.5714, 21.2369)
  line L871 (40.3809, 21.0464) -> (40.3809, 21.4274)
  line L872 (40.1904, 16.9164) -> (40.5714, 16.9164)
  line L873 (40.3809, 16.7259) -> (40.3809, 17.1069)
  line L874 (40.1904, 15.8369) -> (40.5714, 15.8369)
  line L875 (40.3809, 15.6464) -> (40.3809, 16.0274)
  line L876 (41.3156, 15.8369) -> (41.6966, 15.8369)
  line L877 (41.5061, 15.6464) -> (41.5061, 16.0274)
  line L878 (41.3156, 16.9164) -> (41.6966, 16.9164)
  line L879 (41.5061, 16.7259) -> (41.5061, 17.1069)
  line L880 (41.3156, 20.1549) -> (41.6966, 20.1549)
  line L881 (41.5061, 19.9644) -> (41.5061, 20.3454)
  line L882 (41.3156, 19.0754) -> (41.6966, 19.0754)
  line L883 (41.5061, 18.8849) -> (41.5061, 19.2659)
  line L884 (41.3156, 17.9959) -> (41.6966, 17.9959)
  line L885 (41.5061, 17.8054) -> (41.5061, 18.1864)
  line L886 (42.4383, 15.8369) -> (42.8193, 15.8369)
  line L887 (42.6288, 15.6464) -> (42.6288, 16.0274)
  line L888 (42.4383, 16.9164) -> (42.8193, 16.9164)
  line L889 (42.6288, 16.7259) -> (42.6288, 17.1069)
  line L890 (42.4383, 20.1549) -> (42.8193, 20.1549)
  line L891 (42.6288, 19.9644) -> (42.6288, 20.3454)
  line L892 (42.4383, 19.0754) -> (42.8193, 19.0754)
  line L893 (42.6288, 18.8849) -> (42.6288, 19.2659)
  line L894 (42.4383, 17.9959) -> (42.8193, 17.9959)
  line L895 (42.6288, 17.8054) -> (42.6288, 18.1864)
  line L896 (43.5635, 15.8369) -> (43.9445, 15.8369)
  line L897 (43.754, 15.6464) -> (43.754, 16.0274)
  line L898 (43.5635, 16.9164) -> (43.9445, 16.9164)
  line L899 (43.754, 16.7259) -> (43.754, 17.1069)
  line L900 (43.5635, 20.1549) -> (43.9445, 20.1549)
  line L901 (43.754, 19.9644) -> (43.754, 20.3454)
  line L902 (43.5635, 19.0754) -> (43.9445, 19.0754)
  line L903 (43.754, 18.8849) -> (43.754, 19.2659)
  line L904 (43.5635, 17.9959) -> (43.9445, 17.9959)
  line L905 (43.754, 17.8054) -> (43.754, 18.1864)
  line L906 (44.6888, 15.8369) -> (45.0698, 15.8369)
  line L907 (44.8793, 15.6464) -> (44.8793, 16.0274)
  line L908 (44.6888, 16.9164) -> (45.0698, 16.9164)
  line L909 (44.8793, 16.7259) -> (44.8793, 17.1069)
  line L910 (44.6888, 20.1549) -> (45.0698, 20.1549)
  line L911 (44.8793, 19.9644) -> (44.8793, 20.3454)
  line L912 (44.6888, 19.0754) -> (45.0698, 19.0754)
  line L913 (44.8793, 18.8849) -> (44.8793, 19.2659)
  line L914 (44.6888, 17.9959) -> (45.0698, 17.9959)
  line L915 (44.8793, 17.8054) -> (44.8793, 18.1864)
  line L916 (44.6888, 10.6756) -> (45.0698, 10.6756)
  line L917 (44.8793, 10.4851) -> (44.8793, 10.8661)
  line L918 (44.6888, 9.5961) -> (45.0698, 9.5961)
  line L919 (44.8793, 9.4056) -> (44.8793, 9.7866)
  line L920 (44.6888, 8.5166) -> (45.0698, 8.5166)
  line L921 (44.8793, 8.3261) -> (44.8793, 8.7071)
  line L922 (44.6888, 11.7551) -> (45.0698, 11.7551)
  line L923 (44.8793, 11.5646) -> (44.8793, 11.9456)
  line L924 (44.6888, 12.8372) -> (45.0698, 12.8372)
  line L925 (44.8793, 12.6467) -> (44.8793, 13.0277)
  line L926 (43.5635, 10.6756) -> (43.9445, 10.6756)
  line L927 (43.754, 10.4851) -> (43.754, 10.8661)
  line L928 (43.5635, 9.5961) -> (43.9445, 9.5961)
  line L929 (43.754, 9.4056) -> (43.754, 9.7866)
  line L930 (43.5635, 8.5166) -> (43.9445, 8.5166)
  line L931 (43.754, 8.3261) -> (43.754, 8.7071)
  line L932 (43.5635, 11.7551) -> (43.9445, 11.7551)
  line L933 (43.754, 11.5646) -> (43.754, 11.9456)
  line L934 (43.5635, 12.8372) -> (43.9445, 12.8372)
  line L935 (43.754, 12.6467) -> (43.754, 13.0277)
  line L936 (42.4383, 10.6756) -> (42.8193, 10.6756)
  line L937 (42.6288, 10.4851) -> (42.6288, 10.8661)
  line L938 (42.4383, 9.5961) -> (42.8193, 9.5961)
  line L939 (42.6288, 9.4056) -> (42.6288, 9.7866)
  line L940 (42.4383, 8.5166) -> (42.8193, 8.5166)
  line L941 (42.6288, 8.3261) -> (42.6288, 8.7071)
  line L942 (42.4383, 11.7551) -> (42.8193, 11.7551)
  line L943 (42.6288, 11.5646) -> (42.6288, 11.9456)
  line L944 (42.4383, 12.8372) -> (42.8193, 12.8372)
  line L945 (42.6288, 12.6467) -> (42.6288, 13.0277)
  line L946 (41.3156, 10.6756) -> (41.6966, 10.6756)
  line L947 (41.5061, 10.4851) -> (41.5061, 10.8661)
  line L948 (41.3156, 9.5961) -> (41.6966, 9.5961)
  line L949 (41.5061, 9.4056) -> (41.5061, 9.7866)
  line L950 (41.3156, 8.5166) -> (41.6966, 8.5166)
  line L951 (41.5061, 8.3261) -> (41.5061, 8.7071)
  line L952 (41.3156, 11.7551) -> (41.6966, 11.7551)
  line L953 (41.5061, 11.5646) -> (41.5061, 11.9456)
  line L954 (41.3156, 12.8372) -> (41.6966, 12.8372)
  line L955 (41.5061, 12.6467) -> (41.5061, 13.0277)
  line L956 (40.1904, 12.8372) -> (40.5714, 12.8372)
  line L957 (40.3809, 12.6467) -> (40.3809, 13.0277)
  line L958 (40.1904, 11.7551) -> (40.5714, 11.7551)
  line L959 (40.3809, 11.5646) -> (40.3809, 11.9456)
  line L960 (40.1904, 7.4371) -> (40.5714, 7.4371)
  line L961 (40.3809, 7.2466) -> (40.3809, 7.6276)
  line L962 (42.4383, 7.4371) -> (42.8193, 7.4371)
  line L963 (42.6288, 7.2466) -> (42.6288, 7.6276)
  line L964 (40.1904, 8.5166) -> (40.5714, 8.5166)
  line L965 (40.3809, 8.3261) -> (40.3809, 8.7071)
  line L966 (41.3156, 7.4371) -> (41.6966, 7.4371)
  line L967 (41.5061, 7.2466) -> (41.5061, 7.6276)
  line L968 (43.5635, 7.4371) -> (43.9445, 7.4371)
  line L969 (43.754, 7.2466) -> (43.754, 7.6276)
  line L970 (44.6888, 7.4371) -> (45.0698, 7.4371)
  line L971 (44.8793, 7.2466) -> (44.8793, 7.6276)
  line L972 (40.1904, 9.5961) -> (40.5714, 9.5961)
  line L973 (40.3809, 9.4056) -> (40.3809, 9.7866)
  line L974 (40.1904, 10.6756) -> (40.5714, 10.6756)
  line L975 (40.3809, 10.4851) -> (40.3809, 10.8661)
  line L976 (38.5902, 14.9098) -> (38.9712, 14.9098)
  line L977 (38.7807, 14.7193) -> (38.7807, 15.1003)
  line L978 (38.5902, 15.9918) -> (38.9712, 15.9918)
  line L979 (38.7807, 15.8013) -> (38.7807, 16.1823)
  line L980 (37.465, 14.9098) -> (37.846, 14.9098)
  line L981 (37.6555, 14.7193) -> (37.6555, 15.1003)
  line L982 (37.465, 15.9918) -> (37.846, 15.9918)
  line L983 (37.6555, 15.8013) -> (37.6555, 16.1823)